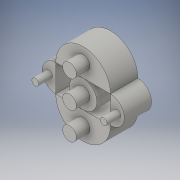
# Autodesk Inventor part: Table
Saved by Autodesk Inventor 2016 (Build 200138000, 138)
## iProperties
Created: 2016-07-18
Part Number: Table
Material: Generic
Document SubType Name: Modeling
Designer: cfkguest
Density: 1 g/cm^3
Appearance: Default
Author: cfkguest
Autodesk Inventor part; units mm, degrees
ref_plane "YZ Plane" through (0, 0, 0) normal (1, 0, 0) x (0, 1, 0)
ref_plane "XZ Plane" through (0, 0, 0) normal (0, 1, 0) x (-1, 0, 0)
ref_plane "XY Plane" through (0, 0, 0) normal (0, 0, 1) x (1, 0, 0)
sketch "Sketch1" plane through (0, 0, 0) normal (0, 0, 1) x (1, 0, 0)
  line L0 (-12.6066, 7.2138) -> (12.7934, 7.2138)
  line L1 (12.7934, 7.2138) -> (12.7934, -5.4862)
  line L2 (12.7934, -5.4862) -> (-12.6066, -5.4862)
  line L3 (-12.6066, -5.4862) -> (-12.6066, 7.2138)
  arc A0 (12.7934, 7.2138) -> (-12.6066, 7.2138) centre (0.0934, 7.2138) ccw
  arc A1 (-12.6066, -5.4862) -> (12.7934, -5.4862) centre (0.0934, -5.4862) ccw
  arc A2 (-12.6066, 7.2138) -> (-12.6066, -5.4862) centre (-12.6066, 0.8638) ccw
  arc A3 (12.7934, -5.4862) -> (12.7934, 7.2138) centre (12.7934, 0.8638) ccw
  circle A4 centre (0.0934, 0.8638) radius 6.35
  point P0 (0, 0)
  dimension "d0" = 12.7
  dimension "d1" = 25.4
  constraints: 8 end point, 8 point on circle, 5 centre point, 4 midpoint, 2 parallel, 1 horizontal, 1 perpendicular
  measures "d0" distance of L2.end L0.start
  measures "d1" distance of L0.start L0.end
extrude "Extrusion1" add sketch "Sketch1" along normal blind 12.7 contours A0 L0 | L3 A2 | A4 | L2 A1 | A3 L1
sketch "Sketch2" plane through (0, 0, 12.7) normal (0, 0, 1) x (1, 0, 0)
  line L0 (0.0934, 7.2138) -> (12.7934, 7.2138) projected
  line L1 (0.0934, 7.2138) -> (0.0934, 13.5638)
  line L2 (12.7934, -5.4862) -> (0.0934, -5.4862) projected
  line L3 (0.0934, -5.4862) -> (0.0934, -11.8362)
  circle A0 centre (0.0934, 13.5638) radius 3.175
  circle A1 centre (0.0934, -11.8362) radius 3.175
  point P0 (0, 0)
  dimension "d4" = 6.35
  dimension "d5" = 6.35
  dimension "d6" = 6.35
  dimension "d7" = 6.35
  constraints: 4 end point, 2 centre point, 2 coincident, 2 vertical
  measures "d4" distance of L0.start L1.end
  measures "d5" distance of L2.end L3.end
  measures "d6" diameter of A0
  measures "d7" diameter of A1
extrude "Extrusion2" add sketch "Sketch2" along normal blind 6.35
sketch "Sketch3" plane through (0, 0, 12.7) normal (0, 0, 1) x (1, 0, 0)
  line L0 (-12.6066, -5.4862) -> (-12.6066, 7.2138) projected
  line L1 (-12.6066, 0.8638) -> (-15.7816, 0.8638)
  line L2 (12.7934, 7.2138) -> (12.7934, -5.4862) projected
  line L3 (12.7934, 0.8638) -> (15.9684, 0.8638)
  circle A0 centre (-15.7816, 0.8638) radius 1.5875
  circle A1 centre (15.9684, 0.8638) radius 1.5875
  point P0 (0, 0)
  dimension "d10" = 3.175
  dimension "d11" = 3.175
  dimension "d12" = 3.175
  dimension "d13" = 3.175
  constraints: 4 end point, 2 centre point, 2 coincident, 2 horizontal, 2 midpoint
  measures "d10" distance of L1.start L1.end
  measures "d11" distance of L3.start L3.end
  measures "d12" diameter of A0
  measures "d13" diameter of A1
extrude "Extrusion3" add sketch "Sketch3" along normal blind 6.35
sketch "Sketch4" plane through (0, 0, 12.7) normal (0, 0, 1) x (1, 0, 0)
  line L0 (-12.6066, 7.2138) -> (0.0934, 7.2138) projected
  arc A0 (0.0934, 7.2138) -> (0.0934, -5.4862) centre (0.0934, 0.8638) ccw projected
  line L1 (0.0934, 7.2138) -> (0.0934, 7.2138)
  arc A1 (0.0934, -5.4862) -> (0.0934, 7.2138) centre (0.0934, 0.8638) ccw projected
  circle A2 centre (0.0934, 0.8638) radius 3.175
  point P0 (0, 0)
  dimension "d16" = 6.35
  constraints: 2 end point, 1 centre point, 1 coincident, 1 perpendicular
  measures "d16" diameter of A2
extrude "Extrusion4" add sketch "Sketch4" along normal blind 6.35 contours A2
body "Solid1"
